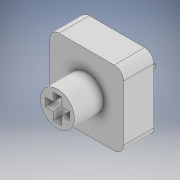
# Autodesk Inventor part: IPC TIME 6 key
Saved by Autodesk Inventor 2022 (Build 260153000, 153)
## iProperties
Created: 2021-12-31
Part Number: IPC TIME 6 key
Material: Generic
Document SubType Name: Modeling
Designer: solor
Density: 1 g/cm^3
Appearance: Default
Author: solor
Autodesk Inventor part; units mm, degrees
ref_plane "YZ Plane" through (0, 0, 0) normal (1, 0, 0) x (0, 1, 0)
ref_plane "XZ Plane" through (0, 0, 0) normal (0, 1, 0) x (-1, 0, 0)
sketch "Sketch1" plane through (0, 0, 0) normal (0, 0, 1) x (1, 0, 0)
  line L0 (14.6962, 12.74) -> (14.6962, 0) construction
  line L1 (10.61, 12.2) -> (1.53, 12.2)
  arc A0 (1.53, 12.2) -> (0, 10.67) centre (1.53, 10.67) ccw
  line L2 (0, 10.67) -> (0, 1.53)
  arc A1 (0, 1.53) -> (1.53, 0) centre (1.53, 1.53) ccw
  line L3 (1.53, 0) -> (10.61, 0)
  arc A2 (10.61, 0) -> (12.14, 1.53) centre (10.61, 1.53) ccw
  arc A3 (12.14, 10.67) -> (10.61, 12.2) centre (10.61, 10.67) ccw
  line L4 (12.14, 10.67) -> (12.14, 1.53)
  point P0 (0, 0)
  point P1 (0, 0)
  dimension "d10" = 12.74
  constraints: 10 end point, 8 point on circle, 4 centre point, 2 vertical, 1 point on line
  measures "d10" distance of L0.start L0.end
ref_plane "Work Plane1" through (0, 0, 5) normal (0, 0, 1) x (1, 0, 0)
sketch "Sketch2" plane through (0, 0, 5) normal (0, 0, 1) x (1, 0, 0)
  line L0 (10.88, 12.74) -> (1.8, 12.74) projected
  line L1 (10.88, 12.74) -> (1.8, 12.74) projected
  arc A0 (1.8, 12.74) -> (0, 10.94) centre (1.8, 10.94) ccw projected
  line L2 (0, 10.94) -> (0, 1.8) projected
  arc A1 (0, 1.8) -> (1.8, 0) centre (1.8, 1.8) ccw projected
  line L3 (1.8, 0) -> (10.88, 0) projected
  arc A2 (10.88, 0) -> (12.68, 1.8) centre (10.88, 1.8) ccw projected
  line L4 (12.68, 1.8) -> (12.68, 10.94) projected
  arc A3 (12.68, 10.94) -> (10.88, 12.74) centre (10.88, 10.94) ccw projected
  circle A4 centre (6.34, 6.37) radius 2.8
  line L5 (5.665, 8.395) -> (7.015, 8.395)
  line L6 (7.015, 4.345) -> (5.665, 4.345)
  line L7 (5.665, 4.345) -> (7.015, 8.395) construction
  line L8 (5.665, 8.395) -> (7.015, 4.345) construction
  line L9 (8.365, 5.695) -> (8.365, 7.045)
  line L10 (4.315, 7.045) -> (4.315, 5.695)
  line L11 (4.315, 5.695) -> (8.365, 7.045) construction
  line L12 (8.365, 5.695) -> (4.315, 7.045) construction
  line L13 (4.315, 5.695) -> (5.665, 5.695)
  line L14 (7.015, 5.695) -> (8.365, 5.695)
  line L15 (5.665, 4.345) -> (5.665, 5.695)
  line L16 (5.665, 7.045) -> (5.665, 8.395)
  line L17 (8.365, 7.045) -> (7.015, 7.045)
  line L18 (5.665, 7.045) -> (4.315, 7.045)
  line L19 (7.015, 8.395) -> (7.015, 7.045)
  line L20 (7.015, 5.695) -> (7.015, 4.345)
  point P0 (0, 0)
  dimension "d3" = 5.6
  dimension "d4" = 4.05
  dimension "d5" = 1.35
  dimension "d6" = 4.05
  dimension "d7" = 1.35
  constraints: 32 end point, 10 parallel, 8 perpendicular, 4 midpoint, 2 vertical, 1 centre point
  measures "d3" diameter of A4
  measures "d4" distance of L6.end L5.start
  measures "d5" distance of L5.start L5.end
  measures "d6" distance of L10.end L9.start
  measures "d7" distance of L9.end L9.start
extrude "Extrusion3" add sketch "Sketch1" along normal blind 5
sketch "Sketch3" plane through (0, 0, 5) normal (0, 0, 1) x (1, 0, 0)
  line L0 (10.61, 12.47) -> (1.53, 12.47)
  line L1 (10.61, 12.47) -> (1.53, 12.47)
  arc A0 (1.53, 12.47) -> (-0.27, 10.67) centre (1.53, 10.67) ccw
  line L2 (-0.27, 10.67) -> (-0.27, 1.53)
  arc A1 (-0.27, 1.53) -> (1.53, -0.27) centre (1.53, 1.53) ccw
  line L3 (1.53, -0.27) -> (10.61, -0.27)
  arc A2 (10.61, -0.27) -> (12.41, 1.53) centre (10.61, 1.53) ccw
  line L4 (12.41, 1.53) -> (12.41, 10.67)
  arc A3 (12.41, 10.67) -> (10.61, 12.47) centre (10.61, 10.67) ccw
  circle A4 centre (6.07, 6.1) radius 2.8
  line L5 (5.395, 8.125) -> (6.745, 8.125)
  line L6 (6.745, 4.075) -> (5.395, 4.075)
  line L7 (5.395, 4.075) -> (6.745, 8.125) construction
  line L8 (5.395, 8.125) -> (6.745, 4.075) construction
  line L9 (8.095, 5.425) -> (8.095, 6.775)
  line L10 (4.045, 6.775) -> (4.045, 5.425)
  line L11 (4.045, 5.425) -> (8.095, 6.775) construction
  line L12 (8.095, 5.425) -> (4.045, 6.775) construction
  line L13 (4.045, 5.425) -> (5.395, 5.425)
  line L14 (6.745, 5.425) -> (8.095, 5.425)
  line L15 (5.395, 4.075) -> (5.395, 5.425)
  line L16 (5.395, 6.775) -> (5.395, 8.125)
  line L17 (8.095, 6.775) -> (6.745, 6.775)
  line L18 (5.395, 6.775) -> (4.045, 6.775)
  line L19 (6.745, 8.125) -> (6.745, 6.775)
  line L20 (6.745, 5.425) -> (6.745, 4.075)
  line L21 (10.61, 12.2) -> (1.53, 12.2) projected
  line L22 (0, 10.67) -> (0, 1.53) projected
  point P0 (0, 0)
  point P1 (-0.27, -0.27)
  point P2 (6.07, 12.2)
  point P3 (0, 6.1)
  point P4 (6.07, 6.1)
  dimension "d14" = 5.6
  dimension "d15" = 4.05
  dimension "d16" = 1.35
  dimension "d17" = 4.05
  dimension "d18" = 1.35
  constraints: 42 end point, 10 parallel, 8 perpendicular, 8 point on circle, 6 midpoint, 5 centre point, 2 vertical
  measures "d14" diameter of A4
  measures "d15" distance of L6.end L5.start
  measures "d16" distance of L5.start L5.end
  measures "d17" distance of L10.end L9.start
  measures "d18" distance of L9.end L9.start
extrude "Extrusion4" add sketch "Sketch3" along normal blind 4.8 contours A4
sketch "Sketch4" plane through (0, 0, 0) normal (0, 0, -1) x (-1, 0, 0)
  line L0 (-13.9436, 0) -> (-13.9436, 2.266)
  line L1 (-15.5559, 0) -> (-15.5559, 6.84)
  line L2 (-1.53, 0) -> (-10.61, 0) projected
  line L3 (-11.5311, 9.89) -> (-0.6089, 9.89) construction
  line L4 (-0.6089, 9.89) -> (-0.6089, 6.84) construction
  line L5 (-0.6089, 6.84) -> (-11.5311, 6.84) construction
  line L6 (-11.5311, 6.84) -> (-11.5311, 9.89) construction
  line L7 (-7.4059, 5.4371) -> (-4.7341, 5.4371) construction
  line L8 (-4.7341, 5.4371) -> (-4.7341, 2.266) construction
  line L9 (-4.7341, 2.266) -> (-7.4059, 2.266) construction
  line L10 (-7.4059, 2.266) -> (-7.4059, 5.4371) construction
  line L11 (-10.6289, 6.84) -> (-10.6289, 9.3092)
  line L12 (-10.6289, 9.3092) -> (-11.5311, 9.3092)
  line L13 (-11.5311, 9.3092) -> (-11.5311, 9.89)
  line L14 (-11.5311, 9.89) -> (-8.9606, 9.89)
  line L15 (-8.9606, 9.89) -> (-8.9606, 9.3092)
  line L16 (-8.9606, 9.3092) -> (-9.8627, 9.3092)
  line L17 (-9.8627, 9.3092) -> (-9.8627, 6.84)
  line L18 (-9.8627, 6.84) -> (-10.6289, 6.84)
  line L19 (-7.1291, 6.84) -> (-8.7703, 6.84)
  line L20 (-8.7703, 6.84) -> (-8.7703, 7.3714)
  line L21 (-8.7703, 7.3714) -> (-8.3328, 7.3714)
  line L22 (-8.3328, 7.3714) -> (-8.3328, 9.3586)
  line L23 (-8.3328, 9.3586) -> (-8.7703, 9.3586)
  line L24 (-8.7703, 9.3586) -> (-8.7703, 9.89)
  line L25 (-8.7703, 9.89) -> (-7.1291, 9.89)
  line L26 (-7.1291, 9.89) -> (-7.1291, 9.3586)
  line L27 (-7.1291, 9.3586) -> (-7.5666, 9.3586)
  line L28 (-7.5666, 9.3586) -> (-7.5666, 7.3714)
  line L29 (-7.5666, 7.3714) -> (-7.1291, 7.3714)
  line L30 (-7.1291, 7.3714) -> (-7.1291, 6.84)
  line L31 (-3.5057, 6.84) -> (-4.2669, 6.84)
  line L32 (-4.2669, 6.84) -> (-4.2669, 8.8618)
  line L33 (-4.2669, 8.8618) -> (-4.8206, 7.5568)
  line L34 (-4.8206, 7.5568) -> (-5.3446, 7.5568)
  line L35 (-5.3446, 7.5568) -> (-5.8982, 8.8618)
  line L36 (-5.8982, 8.8618) -> (-5.8982, 6.84)
  line L37 (-5.8982, 6.84) -> (-6.6199, 6.84)
  line L38 (-6.6199, 6.84) -> (-6.6199, 9.89)
  line L39 (-6.6199, 9.89) -> (-5.7376, 9.89)
  line L40 (-5.7376, 9.89) -> (-5.0603, 8.3848)
  line L41 (-5.0603, 8.3848) -> (-4.3881, 9.89)
  line L42 (-4.3881, 9.89) -> (-3.5057, 9.89)
  line L43 (-3.5057, 9.89) -> (-3.5057, 6.84)
  line L44 (-2.8729, 6.84) -> (-2.8729, 9.89)
  line L45 (-2.8729, 9.89) -> (-0.8116, 9.89)
  line L46 (-0.8116, 9.89) -> (-0.8116, 9.3092)
  line L47 (-0.8116, 9.3092) -> (-2.1117, 9.3092)
  line L48 (-2.1117, 9.3092) -> (-2.1117, 8.7728)
  line L49 (-2.1117, 8.7728) -> (-0.9129, 8.7728)
  line L50 (-0.9129, 8.7728) -> (-0.9129, 8.192)
  line L51 (-0.9129, 8.192) -> (-2.1117, 8.192)
  line L52 (-2.1117, 8.192) -> (-2.1117, 7.4208)
  line L53 (-2.1117, 7.4208) -> (-0.8116, 7.4208)
  line L54 (-0.8116, 7.4208) -> (-0.8116, 6.84)
  line L55 (-0.8116, 6.84) -> (-2.8729, 6.84)
  spline S0 degree 2 poles (-4.8725, 3.3684) (-4.8725, 2.8864) (-5.483, 2.266) (-6.0169, 2.266) knots 0 0 0 1 2 2 2
  spline S1 degree 2 poles (-6.0169, 2.266) (-6.2838, 2.266) (-6.7015, 2.4192) (-6.8473, 2.57) knots 0 0 0 1 2 2 2
  spline S2 degree 2 poles (-6.8473, 2.57) (-7.0203, 2.7455) (-7.2057, 3.3016) (-7.2057, 3.6897) knots 0 0 0 1 2 2 2
  spline S3 degree 2 poles (-7.2057, 3.6897) (-7.2057, 4.0901) (-7.0327, 4.7129) (-6.8374, 4.9527) knots 0 0 0 1 2 2 2
  spline S4 degree 2 poles (-6.8374, 4.9527) (-6.6521, 5.1801) (-6.049, 5.4371) (-5.6362, 5.4371) knots 0 0 0 1 2 2 2
  spline S5 degree 2 poles (-5.6362, 5.4371) (-5.4855, 5.4371) (-5.1839, 5.3976) (-5.1295, 5.3852) knots 0 0 0 1 2 2 2
  line L56 (-5.1295, 5.3852) -> (-5.1295, 4.7871)
  line L57 (-5.1295, 4.7871) -> (-5.1839, 4.7871)
  spline S6 degree 2 poles (-5.1839, 4.7871) (-5.2383, 4.8143) (-5.4855, 4.881) (-5.6436, 4.881) knots 0 0 0 1 2 2 2
  spline S7 degree 2 poles (-5.6436, 4.881) (-6.002, 4.881) (-6.3925, 4.5028) (-6.4395, 4.1519) knots 0 0 0 1 2 2 2
  spline S8 degree 2 poles (-6.4395, 4.1519) (-6.2887, 4.2483) (-5.9798, 4.3619) (-5.7845, 4.3619) knots 0 0 0 1 2 2 2
  spline S9 degree 2 poles (-5.7845, 4.3619) (-5.6189, 4.3619) (-5.3297, 4.273) (-5.2185, 4.1889) knots 0 0 0 1 2 2 2
  spline S10 degree 2 poles (-5.2185, 4.1889) (-5.0603, 4.0678) (-4.8725, 3.6748) (-4.8725, 3.3684) knots 0 0 0 1 2 2 2
  spline S11 degree 2 poles (-5.7648, 2.9086) (-5.7054, 2.9828) (-5.6412, 3.1558) (-5.6412, 3.3313) knots 0 0 0 1 2 2 2
  spline S12 degree 2 poles (-5.6412, 3.3313) (-5.6412, 3.4796) (-5.7153, 3.6724) (-5.7821, 3.7292) knots 0 0 0 1 2 2 2
  spline S13 degree 2 poles (-5.7821, 3.7292) (-5.8513, 3.7885) (-6.0218, 3.8305) (-6.1182, 3.8305) knots 0 0 0 1 2 2 2
  spline S14 degree 2 poles (-6.1182, 3.8305) (-6.1998, 3.8305) (-6.3678, 3.7885) (-6.442, 3.7589) knots 0 0 0 1 2 2 2
  spline S15 degree 2 poles (-6.442, 3.7589) (-6.442, 3.7391) (-6.4469, 3.6452) (-6.4469, 3.5735) knots 0 0 0 1 2 2 2
  spline S16 degree 2 poles (-6.4469, 3.5735) (-6.4469, 3.309) (-6.3555, 2.9902) (-6.2838, 2.9086) knots 0 0 0 1 2 2 2
  spline S17 degree 2 poles (-6.2838, 2.9086) (-6.2319, 2.8419) (-6.0935, 2.785) (-6.0193, 2.785) knots 0 0 0 1 2 2 2
  spline S18 degree 2 poles (-6.0193, 2.785) (-5.9575, 2.785) (-5.8142, 2.8468) (-5.7648, 2.9086) knots 0 0 0 1 2 2 2
  point P0 (0, 0)
  point P1 (-6.07, 0)
  point P2 (-6.07, 2.266)
  point P3 (-6.07, 6.84)
  point P4 (-6.07, 6.84)
  point P5 (-6.07, 2.266)
  dimension "d21" = 2.266
  dimension "d22" = 6.84
  constraints: 4 end point, 3 midpoint, 2 vertical, 4 other
  measures "d21" distance of L0.start L0.end
  measures "d22" distance of L1.start L1.end
extrude "Extrusion5" add sketch "Sketch4" along normal blind 0.9
body "Solid2"
